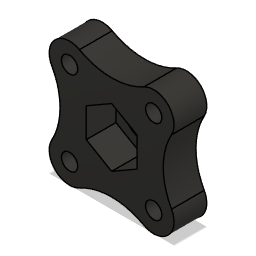
nut retainer v1 (Autodesk Fusion 360 design; units mm, degrees)
Autodesk Fusion 360 part; units mm, degrees
sketch "Sketch1" plane through (0, 0, 0) normal (0, 0, 1) x (1, 0, 0)
  line L0 (-14.1421, 14.1421) -> (14.1421, -14.1421) construction
  line L1 (14.1421, 14.1421) -> (-14.1421, -14.1421) construction
  line L2 (0, 0) -> (-12, 0) construction
  circle A0 centre (14.1421, 14.1421) radius 6.85
  circle A1 centre (-14.1421, 14.1421) radius 6.85
  circle A2 centre (-14.1421, -14.1421) radius 6.85
  circle A3 centre (14.1421, -14.1421) radius 6.85
  line L3 (-17.35, 0) -> (17.35, 0) construction
  arc A4 (-20.14, -10.8333) -> (-20.14, 10.8333) centre (-39.7775, 0) ccw
  arc A5 (-10.8333, 20.14) -> (10.8333, 20.14) centre (0, 39.7775) ccw
  arc A6 (20.14, 10.8333) -> (20.14, -10.8333) centre (39.7775, 0) ccw
  arc A7 (10.8333, -20.14) -> (-10.8333, -20.14) centre (0, -39.7775) ccw
  line L4 (-8.55, -4.9363) -> (0, -9.8727)
  line L5 (0, -9.8727) -> (8.55, -4.9363)
  line L6 (8.55, -4.9363) -> (8.55, 4.9363)
  line L7 (8.55, 4.9363) -> (0, 9.8727)
  line L8 (0, 9.8727) -> (-8.55, 4.9363)
  line L9 (-8.55, 4.9363) -> (-8.55, -4.9363)
  circle A8 centre (-14.1421, 14.1421) radius 2.75
  circle A9 centre (-14.1421, -14.1421) radius 2.75
  circle A10 centre (14.1421, -14.1421) radius 2.75
  circle A11 centre (14.1421, 14.1421) radius 2.75
  circle A12 centre (14.1421, 14.1421) radius 5
  circle A13 centre (14.1421, -14.1421) radius 5
  circle A14 centre (-14.1421, -14.1421) radius 5
  circle A15 centre (-14.1421, 14.1421) radius 5
  circle A16 centre (0, 0) radius 5.5
  dimension "d1" = 45
  dimension "d2" = 40
  dimension "d3" = 13.7
  dimension "d4" = 34.7
  dimension "d5" = 17.1
  dimension "d6" = 5.5
  dimension "d9" = 10
  dimension "d10" = 10
  dimension "d11" = 10
  dimension "d12" = 10
  dimension "d15" = 11
  constraint midpoint L0 L2.start
  constraint midpoint L1 L2.start
  constraint coincident L2.start A16.centre
  constraint horizontal L2
  constraint perpendicular L0 L1
  constraint equal L0 L1
  constraint coincident L1.start A0.centre
  constraint coincident L0.start A1.centre
  constraint coincident L1.end A2.centre
  constraint coincident L0.end A3.centre
  constraint equal A0 A1
  constraint equal A0 A3
  constraint equal A2 A3
  constraint horizontal L3
  constraint midpoint L2.start L3
  constraint coincident L3.start A4
  constraint coincident A2 A4.start
  constraint coincident A1 A4.end
  constraint tangent A1 A4
  constraint tangent A2 A4
  constraint symmetric L0 A4.end A5.start
  constraint symmetric L0 A4.start A5.end
  constraint symmetric L0 A4 A5
  constraint symmetric L1 A4.end A7.start
  constraint symmetric L1 A4.start A7.end
  constraint symmetric L1 A4 A7
  constraint symmetric L1 A5.end A6.start
  constraint symmetric L1 A5.start A6.end
  constraint symmetric L1 A5 A6
  constraint vertical L6
  constraint concentric A1 A8
  constraint concentric A2 A9
  constraint concentric A3 A10
  constraint concentric A0 A11
  constraint equal A8 A11
  constraint equal A10 A11
  constraint equal A9 A10
  constraint concentric A11 A12
  constraint concentric A10 A13
  constraint concentric A9 A14
  constraint concentric A1 A15
  measures "d1" angle of L0 L2
  measures "d2" distance of L0.start L0.end
  measures "d3" diameter of A0
  measures "d4" distance of L3.start L3.end
  measures "d5" distance of L6 L9
  measures "d6" diameter of A8
  measures "d9" diameter of A12
  measures "d10" diameter of A13
  measures "d11" diameter of A14
  measures "d12" diameter of A15
  measures "d15" diameter of A16
extrude "Extrude1" add sketch "Sketch1" along normal blind 11 contours A0 | A0 A1 A2 A3 A4 A5 A6 A7 | A1 | A3 | A2 | A12 | A13 | A14 | A15 makes body 1
extrude "Extrude2" cut sketch "Sketch1" along normal blind 3 contours A12 | A13 | A14 | A15 bodies 1
extrude "Extrude3" add sketch "Sketch1" along normal blind 1 contours L4 L5 L6 L7 L8 L9 bodies 1
sketch "Sketch2" plane through (0, 0, 3) normal (0, 0, -1) x (-1, 0, 0)
  circle A0 centre (-14.1421, 14.1421) radius 2.75
  circle A1 centre (-14.1421, 14.1421) radius 5
  circle A2 centre (-14.1421, -14.1421) radius 2.75
  circle A3 centre (-14.1421, -14.1421) radius 5
  circle A4 centre (14.1421, -14.1421) radius 2.75
  circle A5 centre (14.1421, -14.1421) radius 5
  circle A6 centre (14.1421, 14.1421) radius 2.75
  circle A7 centre (14.1421, 14.1421) radius 5
  line L0 (-16.8921, 18.318) -> (-16.8921, -18.318)
  line L1 (-11.3921, -18.318) -> (-11.3921, 18.318)
  line L2 (-18.318, 16.8921) -> (18.318, 16.8921)
  line L3 (-18.318, 11.3921) -> (18.318, 11.3921)
  line L4 (11.3921, 18.504) -> (11.3921, -18.318)
  line L5 (16.8921, 18.318) -> (16.8921, -18.318)
  line L6 (18.318, -11.3921) -> (-18.318, -11.3921)
  line L7 (18.318, -16.8921) -> (-18.318, -16.8921)
  constraint coincident A1 L0.start
  constraint coincident A3 L0.end
  constraint vertical L0
  constraint coincident A3 L1.start
  constraint coincident A1 L1.end
  constraint parallel L0 L1
  constraint coincident A1 L2.start
  constraint coincident A7 L2.end
  constraint perpendicular L1 L2
  constraint coincident A1 L3.start
  constraint coincident A7 L3.end
  constraint perpendicular L1 L3
  constraint coincident A5 L4.end
  constraint perpendicular L3 L4
  constraint coincident A7 L5.start
  constraint coincident A5 L5.end
  constraint parallel L4 L5
  constraint coincident A5 L6.start
  constraint coincident A3 L6.end
  constraint coincident A5 L7.start
  constraint coincident A3 L7.end
  constraint parallel L6 L7
  constraint perpendicular L5 L6
  constraint tangent A2 L1
  constraint tangent A2 L6
  constraint tangent A2 L0
  constraint tangent A2 L7
  constraint tangent A4 L4
  constraint tangent A4 L5
  constraint tangent A6 L2
  constraint tangent A6 L3
extrude "Extrude4" cut sketch "Sketch2" against normal blind 0.2 contours A0 L1 L3 | A0 L1 L2 | A0 L0 L2 | A1 L0 L1 L2 | A0 L0 L3 | A1 L0 L1 L3 | A3 L0 L1 L6 | A2 L1 L6 | A7 L3 L4 L5 | A6 L3 L4 | A7 L2 L4 L5 | A6 L2 L4 | A2 L0 L6 | A2 L1 L7 | A5 L4 L5 L6 | A6 L3 L5 | A6 L2 L5 | A2 L0 L7 | A4 L4 L6 | A3 L0 L1 L7 | A5 L4 L5 L7 | A4 L4 L7 | A4 L5 L6 | A4 L5 L7 bodies 1
extrude "Extrude5" cut sketch "Sketch2" against normal blind 0.4 contours A0 L1 L3 | A0 L1 L2 | A0 L0 L2 | A0 L0 L3 | A2 L1 L6 | A6 L3 L4 | A6 L2 L4 | A2 L0 L6 | A2 L1 L7 | A6 L3 L5 | A6 L2 L5 | A2 L0 L7 | A4 L4 L6 | A4 L4 L7 | A4 L5 L6 | A4 L5 L7 bodies 1
copy_body "Body->Comp1" bodies 1 removing the originals makes body 2 in component "nut retainer"
component "nut retainer" placed x (1, 0, 0) y (0, 1, 0) z (0, 0, 1) at (0, 0, 0)
named bodies: "nut retainer"
